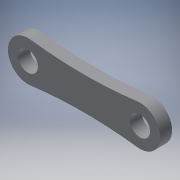
# Autodesk Inventor part: linkageB_mini
Saved by Autodesk Inventor 2017 (Build 210142000, 142)
## iProperties
Created: 2016-08-20
Part Number: linkageB_mini
Material: Generic
Document SubType Name: Modeling
Designer: Nic
Density: 1 g/cm^3
Appearance: Default
Author: Nic
Autodesk Inventor part; units mm, degrees
ref_plane "YZ Plane" through (0, 0, 0) normal (1, 0, 0) x (0, 1, 0)
ref_plane "XZ Plane" through (0, 0, 0) normal (0, 1, 0) x (-1, 0, 0)
ref_plane "XY Plane" through (0, 0, 0) normal (0, 0, 1) x (1, 0, 0)
sketch "Sketch1" plane through (0, 0, 0) normal (0, 0, 1) x (1, 0, 0)
  circle A0 centre (0, 0) radius 1.25
  line L0 (0, 0) -> (14, 0) construction
  circle A1 centre (14, 0) radius 1.25
  arc A2 (0.3211, 2.4793) -> (0.3211, -2.4793) centre (0, 0) ccw
  arc A3 (13.6789, -2.4793) -> (13.6789, 2.4793) centre (14, 0) ccw
  arc A4 (0.3211, 2.4793) -> (13.6789, 2.4793) centre (7, 54.0486) ccw
  arc A5 (13.6789, -2.4793) -> (0.3211, -2.4793) centre (7, -54.0486) ccw
  dimension "d0" = 2.5
  dimension "d1" = 14
  dimension "d8" = 5
  dimension "d15" = 52
  constraints: 8 point on circle, 6 centre point, 4 coincident, 3 symmetric about line, 2 end point, 2 equal radius, 2 tangent, 1 horizontal, 1 other
  measures "d0" diameter of A0
  measures "d1" distance of L0.start L0.end
  measures "d8" diameter of A2
  measures "d15" radius of A4
extrude "Extrusion1" add sketch "Sketch1" along normal blind 1.5
body "Solid1"
